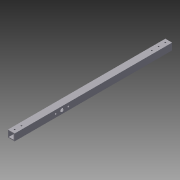
# Autodesk Inventor part: new vertical kicker thing
Saved by Autodesk Inventor 2011 SP1 (Build 150282100, 282)
## iProperties
Created: 2012-01-14
Part Number: new vertical kicker thing
Document SubType Name: Modeling
Designer: Christopher
Density: 1 g/cm^3
Author: Christopher
Autodesk Inventor part; units mm, degrees
ref_plane "YZ Plane" through (0, 0, 0) normal (1, 0, 0) x (0, 1, 0)
ref_plane "XZ Plane" through (0, 0, 0) normal (0, 1, 0) x (-1, 0, 0)
ref_plane "XY Plane" through (0, 0, 0) normal (0, 0, 1) x (1, 0, 0)
sketch "Sketch1" plane through (0, 0, 0) normal (0, 0, 1) x (1, 0, 0)
  line L0 (0, 0) -> (25.4, 0)
  line L1 (25.4, 0) -> (25.4, 25.4)
  line L2 (25.4, 25.4) -> (0, 25.4)
  line L3 (0, 25.4) -> (0, 0)
  line L4 (3.175, 22.225) -> (22.225, 22.225)
  line L5 (22.225, 22.225) -> (22.225, 3.175)
  line L6 (22.225, 3.175) -> (3.175, 3.175)
  line L7 (3.175, 3.175) -> (3.175, 22.225)
  dimension "d0" = 25.4
  dimension "d1" = 25.4
  dimension "d2" = 3.175
  constraints: 16 end point, 4 parallel, 2 perpendicular, 1 horizontal, 3 other
  measures "d0" distance of L1.end L2.end
  measures "d1" distance of L0.end L1.end
  measures "d2" distance between parallel lines of L3 L7
extrude "Extrusion1" add sketch "Sketch1" against normal blind 590.55
sketch "Sketch4" plane through (0, 25.4, 0) normal (0, 1, 0) x (1, 0, 0)
  line L0 (25.4, 590.55) -> (0, 590.55) projected
  line L1 (25.4, 0) -> (0, 0) projected
  point P0 (12.7, 12.7)
  point P1 (12.7, 38.1)
  point P2 (12.7, 577.85)
  point P3 (12.7, 552.45)
  point P4 (12.7, 527.05)
  dimension "d32" = 12.7
  dimension "d33" = 25.4
  dimension "d34" = 12.7
  dimension "d35" = 25.4
  dimension "d36" = 25.4
  measures "d32" distance from line of L1 point (12.7, 12.7)
  measures "d33" distance of point (12.7, 12.7) point (12.7, 38.1)
  measures "d34" distance from line of L0 point (12.7, 577.85)
  measures "d35" distance of point (12.7, 577.85) point (12.7, 552.45)
  measures "d36" distance of point (12.7, 552.45) point (12.7, 527.05)
hole "Hole4" at (12.7, 25.4, -12.7) at (12.7, 25.4, -38.1) at (12.7, 25.4, -577.85) at (12.7, 25.4, -552.45) at (12.7, 25.4, -527.05) direction (0, -1, 0) diameter 5.08 depth 25.4 tip angle 118
sketch "Sketch5" plane through (25.4, 0, 0) normal (1, 0, 0) x (0, 0, -1)
  line L0 (0, 0) -> (0, 25.4) projected
  point P0 (177.8, 12.7)
  point P1 (153.9875, 12.7)
  point P2 (201.6125, 12.7)
  point P3 (0, 12.7)
  dimension "d44" = 23.8125
  dimension "d45" = 23.8125
  dimension "d46" = 177.8
  constraints: 3 horizontal alignment, 1 midpoint
  measures "d44" distance of point (201.613, 12.7) point (177.8, 12.7)
  measures "d45" distance of point (153.988, 12.7) point (177.8, 12.7)
  measures "d46" distance from line of L0 point (177.8, 12.7)
hole "Hole5" at (25.4, 12.7, -153.9875) at (25.4, 12.7, -201.6125) direction (-1, 0, 0) diameter 6.35 depth 25.4 tip angle 118
hole "Hole6" at (25.4, 12.7, -177.8) direction (-1, 0, 0) diameter 12.7 depth 25.4 tip angle 118
body "Solid1"
